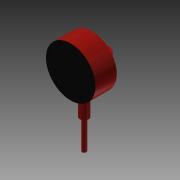
# Autodesk Inventor part: dial-indicator
Saved by Autodesk Inventor 2014 (Build 180170000, 170)
## iProperties
Created: 2013-12-31
Part Number: dial-indicator
Material: Generic
Document SubType Name: Modeling
Designer: caleb
Density: 1 g/cm^3
Appearance: Orange-Red
Author: caleb
Autodesk Inventor part; units mm, degrees
ref_plane "YZ Plane" through (0, 0, 0) normal (1, 0, 0) x (0, 1, 0)
ref_plane "XZ Plane" through (0, 0, 0) normal (0, 1, 0) x (-1, 0, 0)
ref_plane "XY Plane" through (0, 0, 0) normal (0, 0, 1) x (1, 0, 0)
sketch "Sketch2" plane through (0, 0, 0) normal (0, 0, 1) x (1, 0, 0)
  circle A0 centre (0, 0) radius 3.15
  line L0 (-8.5, -10.15) -> (-8.5, 0)
  line L1 (8.5, 0) -> (8.5, -10.15)
  line L2 (-8.5, -10.15) -> (8.5, -10.15)
  arc A1 (8.5, 0) -> (-8.5, 0) centre (0, 0) ccw
  line L3 (0, 8.5) -> (8.5, 8.5) construction
  dimension "d0" = 6.3
  dimension "d1" = 17
  dimension "d2" = 18.65
  constraints: 8 end point, 3 point on circle, 3 tangent, 2 centre point, 2 parallel, 1 coincident, 1 concentric, 1 perpendicular, 1 vertical, 1 vertical alignment
  measures "d0" diameter of A0
  measures "d1" distance between parallel lines of L0 L1
  measures "d2" distance of L3.end L1.end
extrude "Extrusion1" add sketch "Sketch2" along normal blind 6.5
sketch "Sketch3" plane through (-8.5, -10.15, 0) normal (0, -1, 0) x (1, 0, 0)
  line L0 (0, 6.5) -> (17, 6.5) projected
  line L1 (0, 0) -> (0, 6.5) projected
  circle A0 centre (8.5, 3.25) radius 26.7
  point P0 (8.5, 0)
  point P1 (0, 3.25)
  point P2 (0, 3.25)
  point P3 (8.5, 6.5)
  dimension "d5" = 53.4
  constraints: 3 midpoint, 1 centre point, 1 horizontal alignment, 1 vertical alignment
  measures "d5" diameter of A0
extrude "Extrusion2" add sketch "Sketch3" along normal blind 23
sketch "Sketch4" plane through (0, 0, 0) normal (0, 0, -1) x (-1, 0, 0)
  circle A0 centre (0, 0) radius 3.15 projected
  circle A1 centre (0, 0) radius 3.15 projected
  arc A2 (8.5, 0) -> (-8.5, 0) centre (0, 0) ccw projected
  line L0 (8.5, 0) -> (8.5, -10.15) projected
  line L1 (8.5, -10.15) -> (26.5015, -10.15) projected
  line L2 (26.5015, -10.15) -> (26.5015, -33.15) projected
  line L3 (26.5015, -33.15) -> (-26.5015, -33.15) projected
  line L4 (-26.5015, -33.15) -> (-26.5015, -10.15) projected
  line L5 (-26.5015, -10.15) -> (-8.5, -10.15) projected
  line L6 (-8.5, -10.15) -> (8.5, -10.15) projected
  line L7 (-8.5, -10.15) -> (-8.5, 0) projected
  circle A3 centre (0, -18.5) radius 4.76
  dimension "d8" = 9.52
  dimension "d9" = 8.35
  constraints: 1 centre point, 1 vertical alignment
  measures "d8" diameter of A3
  measures "d9" vertical distance of L0.end A3.centre
extrude "Extrusion3" add sketch "Sketch4" along normal blind 46 contours A3
sketch "Sketch5" plane through (0, -18.5, -46) normal (0, 0, -1) x (-1, 0, 0)
  circle A0 centre (0, 0) radius 4.76 projected
  circle A1 centre (0, 0) radius 2.25
  point P0 (0, 18.5)
  dimension "d12" = 4.5
  constraints: 1 centre point, 1 coincident
  measures "d12" diameter of A1
extrude "Extrusion4" add sketch "Sketch5" along normal blind 32 contours A1
body "Solid1"
